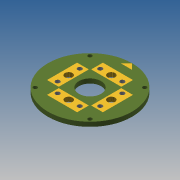
# Autodesk Inventor part: matingBoard
Saved by Autodesk Inventor 2014 SP1 (Build 180222100, 222)
## iProperties
Created: 2014-07-11
Part Number: matingBoard
Material: Generic
Document SubType Name: Modeling
Designer: Dave
Density: 1 g/cm^3
Appearance: Default
Author: Dave
Autodesk Inventor part; units mm, degrees
ref_plane "YZ Plane" through (0, 0, 0) normal (1, 0, 0) x (0, 1, 0)
ref_plane "XZ Plane" through (0, 0, 0) normal (0, 1, 0) x (-1, 0, 0)
ref_plane "XY Plane" through (0, 0, 0) normal (0, 0, 1) x (1, 0, 0)
sketch "Sketch1" plane through (0, 0, 0) normal (0, 1, 0) x (-1, 0, 0)
  circle A0 centre (0, 0.9544) radius 24.13
  point P0 (0, 0)
  dimension "d0" = 48.26
  constraints: 1 centre point
  measures "d0" diameter of A0
extrude "Extrusion1" add sketch "Sketch1" along normal blind 2.54
sketch "Sketch2" plane through (0, 0, 0.9544) normal (0, -1, 0) x (1, 0, 0)
  circle A0 centre (0, 0) radius 24.13 projected
  line L0 (-8.636, 9.3028) -> (8.636, 9.3028)
  line L1 (8.636, 9.3028) -> (8.636, 16.0337)
  line L2 (8.636, 16.0337) -> (-8.636, 16.0337)
  line L3 (-8.636, 16.0337) -> (-8.636, 9.3028)
  line L4 (0, 0) -> (0, 9.3028) construction
  line L5 (0, 9.3028) -> (0, 16.0337) construction
  dimension "d9" = 17.272
  dimension "d10" = 6.731
  dimension "d11" = 9.3027
  constraints: 12 end point, 3 parallel, 2 midpoint, 1 horizontal, 1 perpendicular
  measures "d9" distance of L0.start L0.end
  measures "d10" distance of L2.end L0.start
  measures "d11" distance of L4.start L4.end
extrude "Extrusion2" add sketch "Sketch2" along normal blind 0.0003 and the other way blind 2.5403 contours L3 L2 L1 L0
pattern_circular "Circular Pattern1" count 4 over 360 about axis through (0, 0, 0.9544) along (0, 1, 0) of "Extrusion2"
sketch "Sketch3" plane through (0, 0, 0.9544) normal (0, -1, 0) x (1, 0, 0)
  line L0 (8.636, 9.3027) -> (-8.636, 9.3027) projected
  circle A0 centre (0, 0) radius 24.13 projected
  line L1 (0, 0) -> (15.7154, 15.7154) construction
  line L2 (0, 0) -> (6.7376, 0) construction
  circle A1 centre (15.7154, 15.7154) radius 1.1303
  dimension "d22" = 22.225
  dimension "d23" = 45
  dimension "d24" = 2.2606
  constraints: 4 end point, 1 centre point, 1 coincident, 1 parallel
  measures "d22" distance of L1.start L1.end
  measures "d23" angle of L1 L2
  measures "d24" diameter of A1
hole "Hole1" at (15.7154, 0, 16.6699) direction (0, 1, 0) diameter 2.2606 depth 25.4 tip angle 118
pattern_circular "Circular Pattern2" count 4 over 360 about axis through (0, 0, 0.9544) along (0, 1, 0) of "Hole1"
sketch "Sketch4" plane through (0, -0.0003, 0.9544) normal (0, -1, 0) x (1, 0, 0)
  line L0 (-8.636, 9.3027) -> (8.636, 9.3027) projected
  circle A0 centre (0, 12.2237) radius 1.7579
  point P0 (0, -0.9544)
  dimension "d35" = 2.921
  constraints: 1 centre point
  measures "d35" distance from line of L0 A0.centre
hole "Hole2" at (0, -0.0003, 13.1782) direction (0, 1, 0) diameter 4.2926 depth 25.4 tip angle 118
sketch "Sketch5" plane through (0, -0.0003, 0.9544) normal (0, -1, 0) x (1, 0, 0)
  circle A0 centre (0, 12.2237) radius 2.1463 projected
  line L0 (8.636, 16.0337) -> (-8.636, 16.0337) projected
  circle A1 centre (-6.35, 12.2237) radius 1.1799
  line L1 (0, 12.2237) -> (0, 16.0337) construction
  circle A2 centre (6.35, 12.2237) radius 1.1799
  point P0 (0, -0.9544)
  dimension "d60" = 6.35
  constraints: 2 centre point, 2 end point, 1 midpoint, 1 symmetric about line, 1 other
  measures "d60" distance of A1.centre L1.start
hole "Hole3" at (-6.35, -0.0003, 13.1782) at (6.35, -0.0003, 13.1782) direction (0, 1, 0) diameter 2.54 depth 25.4 tip angle 118
pattern_circular "Circular Pattern3" count 4 over 360 about axis through (0, 0, 0.9544) along (0, 1, 0) of "Hole3", "Hole2"
sketch "Sketch6" plane through (0, 2.54, 0.9544) normal (0, 1, 0) x (1, 0, 0)
  line L0 (8.636, -16.0337) -> (-8.636, -16.0337) projected
  circle A0 centre (0, 0) radius 24.13 projected
  line L1 (0, 24.13) -> (0, 20.828) construction
  line L2 (0, 24.13) -> (3.3047, 20.8253)
  line L3 (0, 24.13) -> (4.6736, 24.13) construction
  line L4 (0, 24.13) -> (-3.3047, 20.8253)
  line L5 (-3.3047, 20.8253) -> (3.3047, 20.8253)
  point P0 (0, 0.9544)
  dimension "d55" = 3.302
  dimension "d56" = 4.6736
  dimension "d57" = 45
  constraints: 10 end point, 1 equal length, 1 horizontal, 1 parallel, 1 perpendicular, 1 symmetric about line, 1 vertical alignment, 1 other
  measures "d55" distance of L1.start L1.end
  measures "d56" distance of L1.start L2.end
  measures "d57" angle of L2 L3
extrude "Extrusion3" add sketch "Sketch6" along normal blind 0.0003 contours L2 L5 L4
sketch "Sketch7" plane through (0, 2.54, 0) normal (0, 1, 0) x (1, 0, 0)
  circle A0 centre (0, -0.9544) radius 24.13 projected
  circle A1 centre (0, -0.9544) radius 6.35
  point P0 (0, 0)
  dimension "d61" = 12.7
  constraints: 1 centre point, 1 coincident
  measures "d61" diameter of A1
hole "Hole4" at (0, 2.54, 0.9544) direction (0, -1, 0) diameter 12.7 depth 25.4 tip angle 118
sketch "Sketch8" plane through (9.3027, -0.0003, -7.6816) normal (0, -1, 0) x (1, 0, 0)
  circle A0 centre (2.921, 8.636) radius 2.1463 projected
sketch "Sketch9" plane through (-16.0337, -0.0003, 9.5904) normal (0, -1, 0) x (1, 0, 0)
  circle A0 centre (3.81, -8.636) radius 2.1463 projected
sketch "Sketch10" plane through (0, -0.0003, 0.9544) normal (0, -1, 0) x (1, 0, 0)
  circle A0 centre (0, 12.2237) radius 2.1463 projected
sketch "Sketch11" plane through (-8.636, -0.0003, -8.3483) normal (0, -1, 0) x (1, 0, 0)
  circle A0 centre (8.636, -2.921) radius 2.1463 projected
body "Solid1"
